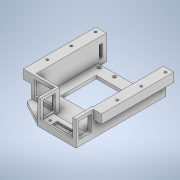
# Autodesk Inventor part: корпус
Saved by Autodesk Inventor 2021.1 (Build 251245010, 245A)
## iProperties
Created: 2021-07-06
Part Number: корпус
Material: Типовые
Document SubType Name: Modeling
Designer: sadmin
Density: 1 g/cm^3
Appearance: По умолчанию
Author: sadmin
Autodesk Inventor part; units mm, degrees
sketch "Эскиз1" plane through (0, 0, 0) normal (0, 0, 1) x (1, 0, 0)
  line L0 (0, 0) -> (84, 0)
  line L1 (84, 0) -> (84, 22)
  line L2 (84, 22) -> (95, 22)
  line L3 (95, 22) -> (95, 34)
  line L4 (95, 34) -> (-11, 34)
  line L5 (-11, 34) -> (-11, 22)
  line L6 (-11, 22) -> (0, 22)
  line L7 (0, 22) -> (0, 0)
  dimension "d0" = 84
  dimension "d1" = 22
  dimension "d2" = 11
  dimension "d3" = 12
  dimension "d4" = 106
  constraints: 16 end point, 4 perpendicular, 2 horizontal, 2 point on line, 1 vertical
  measures "d0" distance of L0.start L0.end
  measures "d1" distance of L0.end L1.end
  measures "d2" distance of L1.end L2.end
  measures "d3" distance of L2.end L3.end
  measures "d4" distance of L3.end L4.end
extrude "Выдавливание1" add sketch "Эскиз1" along normal blind 122
sketch "Эскиз2" plane through (0, 0, 0) normal (0, 0, -1) x (-1, 0, 0)
  line L0 (-84, 0) -> (-84, 22) construction
  line L1 (0, 0) -> (-84, 0) construction
  line L2 (0, 22) -> (0, 0) construction
  line L3 (11, 22) -> (0, 22) construction
  line L4 (11, 34) -> (11, 22) construction
  line L5 (-95, 34) -> (11, 34) construction
  line L6 (-95, 22) -> (-95, 34) construction
  line L7 (-84, 22) -> (-95, 22) construction
  line L8 (-95, 34) -> (11, 34) construction
  line L9 (-80.75, 34) -> (-80.75, 4.2)
  line L10 (-80.75, 4.2) -> (-3.25, 4.2)
  line L11 (-3.25, 4.2) -> (-3.25, 34)
  line L12 (-80.75, 34) -> (-3.25, 34)
  dimension "d7" = 4.2
  dimension "d8" = 14.25
  dimension "d9" = 14.25
  constraints: 8 end point, 2 perpendicular, 2 point on line, 1 collinear, 1 vertical
  measures "d7" distance between parallel lines of L1 L10
  measures "d8" distance between parallel lines of L4 L11
  measures "d9" distance between parallel lines of L6 L9
extrude "Выдавливание2" cut sketch "Эскиз2" against normal blind 95.5
sketch "Эскиз3" plane through (0, 0, 95.5) normal (0, 0, -1) x (-1, 0, 0)
  line L0 (-3.25, 4.2) -> (-80.75, 4.2) construction
  line L1 (-3.25, 34) -> (-3.25, 4.2) construction
  line L2 (-80.75, 34) -> (-3.25, 34) construction
  line L3 (-80.75, 4.2) -> (-80.75, 34) construction
  line L4 (-80.75, 4.2) -> (-80.75, 34) construction
  line L5 (-95, 34) -> (11, 34) construction
  line L6 (-79.75, 34) -> (-79.75, 4.2)
  line L7 (-35.21, 34) -> (-35.21, 4.2)
  line L8 (-79.75, 34) -> (-35.21, 34)
  line L9 (-79.75, 4.2) -> (-35.21, 4.2)
  line L10 (-3.25, 4.2) -> (-80.75, 4.2) construction
  point P0 (0, 0)
  dimension "d12" = 1
  dimension "d13" = 44.54
  constraints: 8 end point, 4 point on line, 2 collinear, 2 perpendicular
  measures "d12" distance between parallel lines of L3 L6
  measures "d13" distance between parallel lines of L7 L6
extrude "Выдавливание3" cut sketch "Эскиз3" against normal blind 8.25
sketch "Эскиз4" plane through (-11, 34, 122) normal (0, 1, 0) x (1, 0, 0)
  line L0 (90.75, 26.5) -> (90.75, 18.25) construction
  line L1 (90.75, 18.25) -> (46.21, 18.25) construction
  line L2 (46.21, 18.25) -> (46.21, 26.5) construction
  line L3 (46.21, 26.5) -> (14.25, 26.5) construction
  line L4 (14.25, 26.5) -> (14.25, 122) construction
  line L5 (14.25, 122) -> (0, 122) construction
  line L6 (0, 122) -> (0, 0) construction
  line L7 (106, 0) -> (0, 0) construction
  line L8 (106, 122) -> (106, 0) construction
  line L9 (106, 122) -> (91.75, 122) construction
  line L10 (91.75, 122) -> (91.75, 26.5) construction
  line L11 (91.75, 26.5) -> (90.75, 26.5) construction
  line L12 (106, 122) -> (106, 0) construction
  line L13 (106, 35.5) -> (0, 35.5) construction
  line L14 (0, 122) -> (0, 0) construction
  line L15 (106, 26.5) -> (0, 26.5) construction
  line L16 (106, 23.5) -> (0, 23.5) construction
  line L17 (43.21, 0) -> (43.21, 23.5)
  line L18 (95, 23.5) -> (95, 0)
  line L19 (43.21, 0) -> (0, 23.5)
  line L20 (95, 0) -> (90.75, 0)
  line L21 (11, 0) -> (95, 0) construction
  line L22 (90.75, 0) -> (90.75, 18.25)
  line L23 (46.21, 18.25) -> (90.75, 18.25) projected
  line L24 (90.75, 18.25) -> (46.21, 18.25)
  line L25 (46.21, 18.25) -> (46.21, 0)
  line L26 (43.21, 0) -> (46.21, 0)
  line L27 (43.21, 23.5) -> (0, 23.5)
  line L28 (95, 23.5) -> (106, 23.5)
  line L29 (106, 23.5) -> (106, 0)
  line L30 (106, 0) -> (95, 0)
  line L31 (43.21, 0) -> (0, 0)
  line L32 (0, 0) -> (0, 23.5)
  line L33 (90.75, 1.75) -> (46.21, 1.75)
  line L34 (90.75, 0) -> (46.21, 0)
  line L35 (79.55, 4.75) -> (57.55, 4.75)
  line L36 (57.55, 4.75) -> (57.55, 11.75)
  line L37 (57.55, 11.75) -> (79.55, 11.75)
  line L38 (79.55, 11.75) -> (79.55, 4.75)
  point P0 (11, 122)
  dimension "d16" = 35.5
  dimension "d17" = 9
  dimension "d18" = 3
  dimension "d19" = 3
  dimension "d20" = 4.25
  dimension "d21" = 1.75
  dimension "d32" = 22
  dimension "d34" = 3
  dimension "d35" = 11.2
  dimension "d36" = 7
  constraints: 46 end point, 14 point on line, 10 perpendicular, 6 collinear, 2 horizontal, 2 parallel, 1 vertical
  measures "d16" distance between parallel lines of L13 L7
  measures "d17" distance between parallel lines of L15 L13
  measures "d18" distance between parallel lines of L16 L15
  measures "d19" distance between parallel lines of L17 L2
  measures "d20" distance between parallel lines of L0 L18
  measures "d21" distance between parallel lines of L21 L33
  measures "d32" distance of L35.start L35.end
  measures "d34" distance between parallel lines of L33 L35
  measures "d35" distance between parallel lines of L22 L38
  measures "d36" distance of L37.end L35.start
extrude "Выдавливание4" cut sketch "Эскиз4" against normal blind 26.8 contours L25 L23 L22 L33 | L35 L36 L37 L38
extrude "Выдавливание5" cut sketch "Эскиз4" against normal blind 35.3 contours L18 L28 L29 L30
extrude "Выдавливание6" cut sketch "Эскиз4" against normal blind 57.55 contours L31 L32 L19
extrude "Выдавливание7" cut sketch "Эскиз4" against normal blind 24.5 contours L25 L33 L22 L34
extrude "Выдавливание8" cut sketch "Эскиз4" against normal up to surface (29.8 mm away) contours L19 L27 L17
extrude "Выдавливание9" cut sketch "Эскиз4" against normal up to surface (29.8 mm away) contours L35 L36 L37 L38
sketch "Эскиз5" plane through (-11, 34, 98.5) normal (0, 0, 1) x (1, 0, 0)
  line L0 (39.21, -5) -> (15, -5)
  line L1 (15, -5) -> (15, -24.8)
  line L2 (15, -24.8) -> (39.21, -24.8)
  line L3 (39.21, -24.8) -> (39.21, -5)
  line L4 (0, 0) -> (43.21, 0) construction
  line L5 (43.21, 0) -> (43.21, -29.8) construction
  line L6 (43.21, -29.8) -> (11, -29.8) construction
  line L7 (11, -29.8) -> (11, -12) construction
  point P0 (11, -34)
  dimension "d39" = 5
  dimension "d40" = 4
  dimension "d41" = 5
  dimension "d42" = 4
  constraints: 8 end point, 2 parallel, 1 horizontal, 1 perpendicular
  measures "d39" distance between parallel lines of L4 L0
  measures "d40" distance between parallel lines of L3 L5
  measures "d41" distance between parallel lines of L6 L2
  measures "d42" distance between parallel lines of L7 L1
extrude "Выдавливание10" cut sketch "Эскиз5" against normal through all
sketch "Эскиз6" plane through (0, 0, 0) normal (0, 0, -1) x (-1, 0, 0)
  line L0 (-3.25, 4.2) -> (-80.75, 4.2) construction
  line L1 (0, 0) -> (-84, 0) construction
  line L2 (-80.75, 4.2) -> (-80.75, 34) construction
  line L3 (-80.75, 4.2) -> (-80.75, 0)
  line L4 (-3.25, 4.2) -> (-3.25, 0)
  line L5 (-80.75, 0) -> (-3.25, 0)
  line L6 (-3.25, 34) -> (-3.25, 4.2) construction
  line L7 (-80.75, 4.2) -> (-3.25, 4.2)
  constraints: 8 end point, 2 perpendicular, 2 point on line, 1 collinear, 1 horizontal
extrude "Выдавливание11" cut sketch "Эскиз6" against normal blind 11.6
sketch "Эскиз7" plane through (-11, 22, 0) normal (0, -1, 0) x (1, 0, 0)
  line L0 (7.1454, 3.15) -> (8.7909, 6)
  line L1 (8.7909, 6) -> (7.1454, 8.85)
  line L2 (2.2091, 6) -> (3.8546, 3.15)
  line L3 (7.1454, 8.85) -> (3.8546, 8.85)
  line L4 (3.8546, 8.85) -> (2.2091, 6)
  line L5 (3.8546, 3.15) -> (7.1454, 3.15)
  circle A0 centre (5.5, 6) radius 1.6
  line L6 (0, 0) -> (11, 0) construction
  line L7 (11, 98.5) -> (0, 98.5) construction
  line L8 (11, 98.5) -> (0, 98.5) construction
  line L9 (0, 0) -> (0, 98.5) construction
  line L10 (0, 0) -> (11, 0) construction
  line L11 (11, 0) -> (11, 98.5) construction
  line L12 (5.5, 0) -> (5.5, 98.5) construction
  line L13 (11, 6) -> (0, 6) construction
  line L14 (0, 0) -> (0, 98.5) construction
  line L15 (11, 0) -> (11, 98.5) construction
  line L16 (11, 39) -> (0, 39) construction
  line L17 (11, 71.5) -> (0, 71.5) construction
  line L18 (7.1454, 41.85) -> (3.8546, 41.85)
  line L19 (8.7909, 39) -> (7.1454, 41.85)
  line L20 (3.8546, 41.85) -> (2.2091, 39)
  circle A1 centre (5.5, 39) radius 1.6
  line L21 (7.1454, 36.15) -> (8.7909, 39)
  line L22 (3.8546, 36.15) -> (7.1454, 36.15)
  line L23 (2.2091, 39) -> (3.8546, 36.15)
  line L24 (7.1454, 74.35) -> (3.8546, 74.35)
  line L25 (8.7909, 71.5) -> (7.1454, 74.35)
  line L26 (3.8546, 74.35) -> (2.2091, 71.5)
  circle A2 centre (5.5, 71.5) radius 1.6
  line L27 (7.1454, 68.65) -> (8.7909, 71.5)
  line L28 (3.8546, 68.65) -> (7.1454, 68.65)
  line L29 (2.2091, 71.5) -> (3.8546, 68.65)
  line L30 (53, -58.192) -> (53, 154.452)
  line L31 (98.8546, 8.85) -> (102.1454, 8.85)
  line L32 (97.2091, 6) -> (98.8546, 8.85)
  line L33 (102.1454, 8.85) -> (103.7909, 6)
  circle A3 centre (100.5, 6) radius 1.6
  line L34 (98.8546, 3.15) -> (97.2091, 6)
  line L35 (102.1454, 3.15) -> (98.8546, 3.15)
  line L36 (103.7909, 6) -> (102.1454, 3.15)
  line L37 (98.8546, 41.85) -> (102.1454, 41.85)
  line L38 (102.1454, 41.85) -> (103.7909, 39)
  line L39 (97.2091, 39) -> (98.8546, 41.85)
  line L40 (103.7909, 39) -> (102.1454, 36.15)
  line L41 (98.8546, 36.15) -> (97.2091, 39)
  circle A4 centre (100.5, 39) radius 1.6
  line L42 (102.1454, 36.15) -> (98.8546, 36.15)
  line L43 (98.8546, 74.35) -> (102.1454, 74.35)
  line L44 (102.1454, 74.35) -> (103.7909, 71.5)
  line L45 (97.2091, 71.5) -> (98.8546, 74.35)
  line L46 (103.7909, 71.5) -> (102.1454, 68.65)
  line L47 (98.8546, 68.65) -> (97.2091, 71.5)
  circle A5 centre (100.5, 71.5) radius 1.6
  line L48 (102.1454, 68.65) -> (98.8546, 68.65)
  point P0 (5.5, 6)
  point P1 (100.5, 6)
  dimension "d47" = 120
  dimension "d48" = 120
  dimension "d49" = 5.7
  dimension "d50" = 3.2
  dimension "d51" = 5.5
  dimension "d52" = 6
  dimension "d53" = 33
  dimension "d54" = 32.5
  dimension "d55" = 120
  dimension "d56" = 120
  dimension "d57" = 5.7
  dimension "d58" = 3.2
  dimension "d59" = 120
  dimension "d60" = 120
  dimension "d61" = 5.7
  dimension "d62" = 3.2
  dimension "d63" = 106
  constraints: 82 end point, 25 symmetric about line, 15 equal length, 6 centre point, 6 point on line, 5 coincident, 5 midpoint, 4 horizontal, 4 parallel, 2 perpendicular, 1 vertical, 3 other
  measures "d47" angle of L5 L2
  measures "d48" angle of L4 L2
  measures "d49" distance between parallel lines of L3 L5
  measures "d50" diameter of A0
  measures "d51" distance between parallel lines of L9 L12
  measures "d52" distance between parallel lines of L6 L13
  measures "d53" distance between parallel lines of L13 L16
  measures "d54" distance between parallel lines of L17 L16
  measures "d55" angle of L22 L23
  measures "d56" angle of L20 L23
  measures "d57" distance between parallel lines of L18 L22
  measures "d58" diameter of A1
  measures "d59" angle of L28 L29
  measures "d60" angle of L26 L29
  measures "d61" distance between parallel lines of L24 L28
  measures "d62" diameter of A2
  measures "d63" diameter of L9 L30
extrude "Выдавливание12" cut sketch "Эскиз7" against normal through all contours A0 | A1 | A2 | A3 | A4 | A5
extrude "Выдавливание13" cut sketch "Эскиз7" against normal blind 3 contours L5 L2 L4 L3 L1 L0 | L19 L21 L22 L23 L20 L18 | L25 L27 L28 L29 L26 L24 | A2 | L31 L33 L36 L35 L34 L32 | A3 | L37 L38 L40 L42 L41 L39 | A4 | L43 L44 L46 L48 L47 L45
sketch "Эскиз8" plane through (32.21, 34, 98.5) normal (-1, 0, 0) x (0, 0, 1)
  line L0 (3, -4) -> (19.5, -4)
  line L1 (19.5, -4) -> (19.5, -25.8)
  line L2 (19.5, -25.8) -> (3, -25.8)
  line L3 (3, -25.8) -> (3, -4)
  line L4 (23.5, -29.8) -> (0, -29.8) construction
  line L5 (23.5, 0) -> (23.5, -29.8) construction
  line L6 (0, 0) -> (23.5, 0) construction
  line L7 (0, 0) -> (0, -29.8) construction
  point P0 (-98.5, -34)
  dimension "d68" = 4
  dimension "d69" = 3
  dimension "d70" = 4
  dimension "d71" = 4
  constraints: 8 end point, 2 parallel, 1 horizontal, 1 perpendicular
  measures "d68" distance between parallel lines of L6 L0
  measures "d69" distance between parallel lines of L7 L3
  measures "d70" distance between parallel lines of L5 L1
  measures "d71" distance between parallel lines of L2 L4
extrude "Выдавливание14" cut sketch "Эскиз8" against normal through all
sketch "Эскиз9" plane through (35.21, 4.2, 103.75) normal (0, 1, 0) x (1, 0, 0)
  line L0 (-18.96, 77.15) -> (32.54, 77.15)
  line L1 (32.54, 77.15) -> (32.54, 28.25)
  line L2 (32.54, 28.25) -> (-18.96, 28.25)
  line L3 (-18.96, 28.25) -> (-18.96, 77.15)
  line L4 (45.54, 92.15) -> (-31.96, 92.15) construction
  line L5 (-31.96, 92.15) -> (-31.96, 8.25) construction
  line L6 (-31.96, 8.25) -> (0, 8.25) construction
  line L7 (0, 8.25) -> (0, 0) construction
  line L8 (0, 0) -> (44.54, 0) construction
  line L9 (44.54, 8.25) -> (44.54, 0) construction
  line L10 (44.54, 8.25) -> (45.54, 8.25) construction
  line L11 (45.54, 92.15) -> (45.54, 8.25) construction
  point P0 (-35.21, 103.75)
  dimension "d74" = 15
  dimension "d75" = 13
  dimension "d76" = 20
  dimension "d77" = 13
  constraints: 8 end point, 2 parallel, 1 horizontal, 1 perpendicular
  measures "d74" distance between parallel lines of L4 L0
  measures "d75" distance between parallel lines of L3 L5
  measures "d76" distance between parallel lines of L2 L6
  measures "d77" distance between parallel lines of L1 L11
extrude "Выдавливание15" cut sketch "Эскиз9" against normal through all
sketch "Эскиз10" plane through (-11, 7.2, 122) normal (0, 1, 0) x (1, 0, 0)
  circle A0 centre (52.15, 7.75) radius 1.6 projected
  circle A1 centre (85.25, 7.75) radius 1.6 projected
  point P0 (11, 122)
extrude "Выдавливание16" cut sketch "Эскиз10" against normal through all
sketch "Эскиз11" plane through (84, 0, 0) normal (0, -1, 0) x (1, 0, 0)
  circle A0 centre (-9.75, 114.25) radius 1.6 construction
  circle A1 centre (-42.85, 114.25) radius 1.6 construction
  line L0 (-16.25, 75.5) -> (-16.25, 26.6) construction
  line L1 (-16.25, 26.6) -> (-67.75, 26.6) construction
  line L2 (-67.75, 26.6) -> (-67.75, 75.5) construction
  line L3 (-67.75, 75.5) -> (-16.25, 75.5) construction
  line L4 (-80.75, 0) -> (-80.75, 11.6) construction
  line L5 (-80.75, 11.6) -> (-3.25, 11.6) construction
  line L6 (-3.25, 11.6) -> (-3.25, 0) construction
  line L7 (-84, 0) -> (-80.75, 0) construction
  line L8 (0, 0) -> (0, 122) construction
  line L9 (-51.79, 122) -> (0, 122) construction
  line L10 (-51.79, 122) -> (-84, 104.4824) construction
  line L11 (-84, 0) -> (-84, 104.4824) construction
  line L12 (-3.25, 0) -> (0, 0) construction
  line L13 (-4.5, 11.6) -> (-34.65, 11.6)
  line L14 (-34.65, 11.6) -> (-34.65, 19.1)
  line L15 (-34.65, 19.1) -> (-4.5, 19.1)
  line L16 (-4.5, 19.1) -> (-4.5, 11.6)
  line L17 (-80.75, 11.6) -> (-3.25, 11.6) construction
  circle A2 centre (-9.05, 15.85) radius 1.35
  circle A3 centre (-30.1, 15.85) radius 1.35
  line L18 (-42, -14.4587) -> (-42, 143.3531)
  line L19 (-95, 0) -> (-95, 98.5) construction
  line L20 (-79.5, 11.6) -> (-49.35, 11.6)
  line L21 (-49.35, 11.6) -> (-49.35, 19.1)
  line L22 (-49.35, 19.1) -> (-79.5, 19.1)
  line L23 (-79.5, 19.1) -> (-79.5, 11.6)
  circle A4 centre (-74.95, 15.85) radius 1.35
  circle A5 centre (-53.9, 15.85) radius 1.35
  dimension "d82" = 4.5
  dimension "d83" = 7.5
  dimension "d84" = 30.15
  dimension "d85" = 2.7
  dimension "d86" = 2.7
  dimension "d87" = 21.05
  dimension "d88" = 4.55
  dimension "d89" = 4.25
  dimension "d91" = 4.25
  dimension "d92" = 106
  constraints: 18 end point, 6 symmetric about line, 4 centre point, 2 parallel, 1 collinear, 1 horizontal, 1 perpendicular, 1 vertical, 2 other
  measures "d82" distance between parallel lines of L8 L16
  measures "d83" distance between parallel lines of L5 L15
  measures "d84" distance between parallel lines of L14 L16
  measures "d85" diameter of A2
  measures "d86" diameter of A3
  measures "d87" distance of A3.centre A2.centre
  measures "d88" distance from line of L16 A2.centre
  measures "d89" distance from line of L5 A2.centre
  measures "d91" distance from line of L17 A3.centre
  measures "d92" diameter of L19 L18
extrude "Выдавливание17" cut sketch "Эскиз11" against normal through all contours A2 | A3 | A4 | A5
extrude "Выдавливание18" cut sketch "Эскиз11" against normal blind 1
sketch "Эскиз12" plane through (84, 0, 0) normal (0, -1, 0) x (1, 0, 0)
  circle A0 centre (-9.75, 114.25) radius 1.6 construction
  circle A1 centre (-42.85, 114.25) radius 1.6 construction
  line L0 (-13.2536, 112.045) -> (-13.4114, 116.1817)
  line L1 (-13.4114, 116.1817) -> (-9.9078, 118.3867)
  line L2 (-9.9078, 118.3867) -> (-6.2464, 116.455)
  line L3 (-6.2464, 116.455) -> (-6.0886, 112.3183)
  line L4 (-6.0886, 112.3183) -> (-9.5922, 110.1133)
  line L5 (-9.5922, 110.1133) -> (-13.2536, 112.045)
  line L6 (-38.6812, 111.4994) -> (-43.1477, 109.2644)
  line L7 (-43.1477, 109.2644) -> (-47.3165, 112.015)
  line L8 (-47.3165, 112.015) -> (-47.0188, 117.0006)
  line L9 (-47.0188, 117.0006) -> (-42.5523, 119.2356)
  line L10 (-42.5523, 119.2356) -> (-38.3835, 116.485)
  line L11 (-38.3835, 116.485) -> (-38.6812, 111.4994)
  line L12 (-51.79, 122) -> (0, 122) construction
  point P0 (-84, 0)
  constraints: 24 end point, 2 coincident, 26 other
extrude "Выдавливание19" cut sketch "Эскиз12" against normal blind 3
ref_plane "РабПлоскость1" through (42, 0, 0) normal (-1, 0, 0) x (0, 0, 1)
sketch "Эскиз14" plane through (3.25, 0, 0) normal (1, 0, 0) x (0, 0, -1)
  line L0 (-9.24, 24.5) -> (-6.24, 24.5) construction
  line L1 (-9.24, 8.5) -> (-6.24, 8.5) construction
  line L2 (-6.24, 24.5) -> (-6.24, 8.5) construction
  line L3 (-9.24, 24.5) -> (-9.24, 8.5) construction
  line L4 (-5.74, 8) -> (-9.74, 8)
  line L5 (-9.74, 8) -> (-9.74, 25)
  line L6 (-9.74, 25) -> (-5.74, 25)
  line L7 (-5.74, 25) -> (-5.74, 8)
  point P0 (0, 0)
  dimension "d103" = 0.5
  constraints: 12 end point, 2 perpendicular, 3 other
  measures "d103" distance between parallel lines of L2 L7
sketch "Эскиз15" plane through (80.75, 0, 0) normal (-1, 0, 0) x (0, 0, 1)
  line L0 (9.24, 24.5) -> (6.24, 24.5) construction
  line L1 (9.24, 8.5) -> (6.24, 8.5) construction
  line L2 (6.24, 24.5) -> (6.24, 8.5) construction
  line L3 (9.24, 24.5) -> (9.24, 8.5) construction
  line L4 (5.74, 8) -> (9.74, 8)
  line L5 (9.74, 8) -> (9.74, 25)
  line L6 (9.74, 25) -> (5.74, 25)
  line L7 (5.74, 25) -> (5.74, 8)
  point P0 (0, 0)
  dimension "d106" = 0.5
  constraints: 12 end point, 2 parallel, 2 perpendicular, 3 other
  measures "d106" distance between parallel lines of L2 L7
extrude "Выдавливание20" cut sketch "Эскиз14" against normal blind 3
extrude "Выдавливание21" cut sketch "Эскиз15" against normal blind 3
sketch "Эскиз16" plane through (35.21, 4.2, 103.75) normal (0, 1, 0) x (1, 0, 0)
  circle A0 centre (-26.16, 87.9) radius 1.35 construction
  circle A1 centre (-5.11, 87.9) radius 1.35 construction
  circle A2 centre (18.69, 87.9) radius 1.35 construction
  circle A3 centre (39.74, 87.9) radius 1.35 construction
  point P0 (-35.21, 103.75)
ref_plane "РабПлоскость2" through (9.05, 4.2, 15.85) normal (1, 0, 0) x (0, 0, -1)
ref_plane "РабПлоскость3" through (30.1, 4.2, 15.85) normal (1, 0, 0) x (0, 0, -1)
ref_plane "РабПлоскость4" through (42, 0, 0) normal (1, 0, 0) x (0, 0, -1)
sketch "Эскиз17" plane through (9.05, 4.2, 15.85) normal (1, 0, 0) x (0, 0, -1)
  line L0 (7.6917, -2.2286) -> (7.6917, 0.2714)
  line L1 (10.7924, -2.1286) -> (3.8592, -2.1286) construction
  line L2 (7.6917, 0.2714) -> (5.2917, -2.1286)
  line L3 (7.6917, -0.7786) -> (6.6417, -0.7786)
  line L4 (4.4917, -0.7786) -> (7.6917, -0.7786) construction
  line L5 (0, 2.965) -> (0, -10.627)
  line L6 (0, 0) -> (-2.45, 0)
  line L7 (4.25, 0) -> (-79.65, 0) projected
  line L8 (-2.45, 0) -> (0, -2.45)
  point P0 (15.85, -4.2)
  point P1 (7.6917, -0.7786)
  point P2 (7.6917, -2.1286)
  point P3 (6.0917, -2.1286)
  point P4 (6.0917, -1.3286)
  point P5 (4.4917, -2.1286)
  point P6 (4.4917, -2.1286)
  dimension "d109" = 4.8
  dimension "d110" = 1.05
  dimension "d111" = 2.45
  dimension "d112" = 45
  dimension "d113" = 45
  constraints: 16 end point, 10 point on line, 2 horizontal, 1 vertical
  measures "d109" diameter of L0.end L1
  measures "d110" distance of L3.start L3.end
  measures "d111" distance of L6.start L6.end
  measures "d112" angle of L0 L2
  measures "d113" angle of L6 L8
revolve "Вращение1" cut sketch "Эскиз17" angle 360 about axis through (9.05, 7.165, 15.85) along (0, -1, 0) contours L5 L8 L6
sketch "Эскиз18" plane through (30.1, 0, 0) normal (1, 0, 0) x (0, 0, -1)
  line L0 (-17.2, 4.2) -> (-14.5, 4.2) construction
  line L1 (-15.85, -1.0746) -> (-15.85, 5.5754)
  line L2 (-15.85, 4.2) -> (-18.3, 4.2)
  line L3 (-18.3, 4.2) -> (-13.4, 4.2) projected
  line L4 (-18.3, 4.2) -> (-15.85, 1.75)
  point P0 (0, 0)
  dimension "d116" = 45
  dimension "d117" = 4.9
  constraints: 6 end point, 2 point on line, 1 horizontal, 1 midpoint, 1 vertical
  measures "d116" angle of L2 L4
  measures "d117" diameter of L2.end L1
revolve "Вращение2" cut sketch "Эскиз18" angle 360 about axis through (30.1, -1.0746, 15.85) along (0, 1, 0)
mirror "Зеркальное отражение1" about plane through (42, 0, 0) normal (1, 0, 0) of "Вращение1", "Вращение2"
